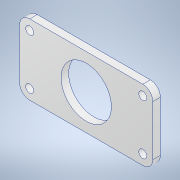
# Autodesk Inventor part: 関節3_プーリ側板
Saved by Autodesk Inventor 2021 (Build 250183000, 183)
## iProperties
Created: 2022-02-02
Part Number: 関節3_プーリ側板
Material: アルミニウム 6061
Document SubType Name: Modeling
Designer: hirohumi
Density: 2.7 g/cm^3
Appearance: アルミニウム - フラット
Author: hirohumi
Autodesk Inventor part; units mm, degrees
ref_plane "YZ Plane" through (0, 0, 0) normal (1, 0, 0) x (0, 1, 0)
ref_plane "XZ Plane" through (0, 0, 0) normal (0, 1, 0) x (-1, 0, 0)
ref_plane "XY Plane" through (0, 0, 0) normal (0, 0, 1) x (1, 0, 0)
sketch "スケッチ1" plane through (0, 0, 0) normal (0, 0, 1) x (1, 0, 0)
  circle A0 centre (0, 0) radius 10
  line L0 (22.5, 10) -> (-22.5, 10) construction
  line L1 (-22.5, 10) -> (-22.5, -10) construction
  line L2 (-22.5, -10) -> (22.5, -10) construction
  line L3 (22.5, -10) -> (22.5, 10) construction
  line L4 (22.5, 10) -> (-22.5, -10) construction
  line L5 (-22.5, 10) -> (22.5, -10) construction
  circle A1 centre (-22.5, 10) radius 1.6
  circle A2 centre (-22.5, -10) radius 1.6
  circle A3 centre (22.5, 10) radius 1.6
  circle A4 centre (22.5, -10) radius 1.6
  line L6 (26.5, 14) -> (-26.5, 14)
  line L7 (-26.5, 14) -> (-26.5, -14)
  line L8 (-26.5, -14) -> (26.5, -14)
  line L9 (26.5, -14) -> (26.5, 14)
  line L10 (26.5, 14) -> (-26.5, -14) construction
  line L11 (-26.5, 14) -> (26.5, -14) construction
  dimension "d0" = 20
  dimension "d1" = 45
  dimension "d2" = 20
  dimension "d3" = 3.2
  dimension "d4" = 3.2
  dimension "d5" = 3.2
  dimension "d6" = 3.2
  dimension "d7" = 4
  dimension "d8" = 4
  constraints: 24 end point, 5 centre point, 5 coincident, 4 midpoint, 4 parallel, 2 horizontal, 2 perpendicular
  measures "d0" diameter of A0
  measures "d1" distance of L2.end L1.end
  measures "d2" distance of L1.end L0.end
  measures "d3" diameter of A1
  measures "d4" diameter of A2
  measures "d5" diameter of A3
  measures "d6" diameter of A4
  measures "d7" distance from line of L0.end L6
  measures "d8" distance from line of L1.end L7
extrude "押し出し1" add sketch "スケッチ1" along normal blind 3
fillet "フィレット1" radius 4 4 edges at (-26.5, 14, 1.5) (26.5, 14, 1.5) (26.5, -14, 1.5) (-26.5, -14, 1.5)
